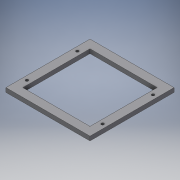
# Autodesk Inventor part: Smooth Rod Brace Bottom
Saved by Autodesk Inventor 2016 (Build 200138000, 138)
## iProperties
Created: 2017-05-17
Part Number: Smooth Rod Brace Bottom
Material: Generic
Document SubType Name: Modeling
Designer: 31745
Density: 1 g/cm^3
Appearance: Default
Author: 31745
Autodesk Inventor part; units mm, degrees
ref_plane "YZ Plane" through (0, 0, 0) normal (1, 0, 0) x (0, 1, 0)
ref_plane "XZ Plane" through (0, 0, 0) normal (0, 1, 0) x (-1, 0, 0)
ref_plane "XY Plane" through (0, 0, 0) normal (0, 0, 1) x (1, 0, 0)
sketch "Sketch1" plane through (0, 0, 0) normal (0, 1, 0) x (-1, 0, 0)
  line L0 (0, 0) -> (-254, 0)
  line L1 (-254, 0) -> (-254, -254)
  line L2 (-254, -254) -> (0, -254)
  line L3 (0, -254) -> (0, 0)
  line L4 (-25.4, -228.6) -> (-228.6, -228.6)
  line L5 (-228.6, -228.6) -> (-228.6, -25.4)
  line L6 (-228.6, -25.4) -> (-25.4, -25.4)
  line L7 (-25.4, -25.4) -> (-25.4, -228.6)
  point P0 (-127, -228.6)
  point P1 (-127, -254)
  point P2 (-228.6, -127)
  point P3 (-254, -127)
  dimension "d0" = 254
  dimension "d1" = 254
  dimension "d2" = 25.4
  dimension "d3" = 25.4
  constraints: 16 end point, 4 midpoint, 4 parallel, 2 horizontal, 2 perpendicular, 1 horizontal alignment, 1 vertical alignment
  measures "d0" distance of L2.end L1.end
  measures "d1" distance of L1.end L0.end
  measures "d2" distance between parallel lines of L2 L4
  measures "d3" distance between parallel lines of L1 L5
extrude "Extrusion1" add sketch "Sketch1" along normal blind 12.7
sketch "Sketch2" plane through (0, 12.7, 0) normal (0, 1, 0) x (1, 0, 0)
  line L0 (0, 254) -> (0, 0) projected
  line L1 (254, 0) -> (254, 254) projected
  line L2 (25.4, 228.6) -> (228.6, 228.6) projected
  line L3 (228.6, 25.4) -> (25.4, 25.4) projected
  point P0 (12.7, 50.8)
  point P1 (12.7, 203.2)
  point P2 (241.3, 203.2)
  point P3 (241.3, 50.8)
  dimension "d6" = 12.7
  dimension "d7" = 12.7
  dimension "d8" = 25.4
  dimension "d9" = 25.4
  constraints: 2 horizontal alignment, 2 vertical alignment
  measures "d6" distance from line of L0 point (12.7, 203.2)
  measures "d7" distance from line of L1 point (241.3, 203.2)
  measures "d8" distance from line of point (12.7, 203.2) L2
  measures "d9" distance from line of L3 point (12.7, 50.8)
hole "Hole1" at (12.7, 12.7, -50.8) at (12.7, 12.7, -203.2) at (241.3, 12.7, -203.2) at (241.3, 12.7, -50.8) direction (0, -1, 0) diameter 8.4074 end through all clearance for "Countersunk Flat Head Screw ISO 2009/7046" size "M8" standard "ISO"
equation "\"d7\" = d6"
equation "\"d9\" = d8"
body "Solid1"
